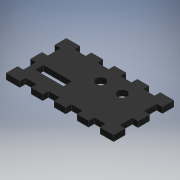
# Autodesk Inventor part: left
Saved by Autodesk Inventor 2019 (Build 230136000, 136)
## iProperties
Created: 2018-06-07
Part Number: left
Material: PBT Plastic Black
Document SubType Name: Modeling
Designer: stra92745
Density: 1.31 g/cm^3
Appearance: Smooth - White
Author: stra92745
Autodesk Inventor part; units mm, degrees
ref_plane "YZ Plane" through (0, 0, 0) normal (1, 0, 0) x (0, 1, 0)
ref_plane "XZ Plane" through (0, 0, 0) normal (0, 1, 0) x (-1, 0, 0)
ref_plane "XY Plane" through (0, 0, 0) normal (0, 0, 1) x (1, 0, 0)
sketch "Sketch1" plane through (0, 0, 0) normal (0, 1, 0) x (-1, 0, 0)
  line L0 (0, 0) -> (-75, 0)
  line L1 (-75, 0) -> (-75, -42)
  line L2 (-75, -42) -> (0, -42)
  line L3 (0, -42) -> (0, 0)
  line L4 (-8, -18) -> (-28, -18)
  line L5 (-28, -18) -> (-28, -12)
  line L6 (-28, -12) -> (-8, -12)
  line L7 (-8, -12) -> (-8, -18)
  circle A0 centre (-38, -28) radius 3.5
  circle A1 centre (-53, -28) radius 3.5
  dimension "d0" = 75
  dimension "d1" = 42
  dimension "d2" = 20
  dimension "d3" = 6
  dimension "d4" = 12
  dimension "d5" = 8
  dimension "d6" = 7
  dimension "d7" = 28
  dimension "d8" = 38
  dimension "d9" = 15
  constraints: 16 end point, 4 parallel, 2 centre point, 2 horizontal, 2 perpendicular, 1 equal radius, 1 horizontal alignment
  measures "d0" distance of L2.end L1.end
  measures "d1" distance of L1.end L0.end
  measures "d2" distance of L4.start L4.end
  measures "d3" distance of L4.end L5.end
  measures "d4" distance between parallel lines of L0 L6
  measures "d5" distance between parallel lines of L3 L7
  measures "d6" diameter of A0
  measures "d7" distance from line of L0 A0.centre
  measures "d8" distance from line of L3 A0.centre
  measures "d9" distance of A1.centre A0.centre
extrude "Extrusion1" add sketch "Sketch1" along normal blind 4
sketch "Sketch2" plane through (0, 4, 0) normal (0, 1, 0) x (1, 0, 0)
  line L0 (0, 42) -> (0, 0) construction
  line L1 (75, 42) -> (0, 42) construction
  line L2 (75, 0) -> (75, 42) construction
  line L3 (0, 0) -> (75, 0) construction
  line L4 (4, 38) -> (4, 4) construction
  line L5 (4, 4) -> (71, 4) construction
  line L6 (71, 4) -> (71, 38) construction
  line L7 (71, 38) -> (4, 38) construction
  line L8 (0, 42) -> (0, 0) construction
  line L9 (0, 21) -> (75, 21) construction
  line L10 (37.5, 42) -> (37.5, 0) construction
  line L11 (0, 34) -> (4, 34)
  line L12 (4, 34) -> (4, 25)
  line L13 (4, 25) -> (0, 25)
  line L14 (0, 25) -> (0, 34)
  line L15 (75, 42) -> (0, 42) projected
  line L16 (9.5, 38) -> (17.5, 38)
  line L17 (17.5, 38) -> (17.5, 42)
  line L18 (17.5, 42) -> (9.5, 42)
  line L19 (9.5, 42) -> (9.5, 38)
  line L20 (25.5, 38) -> (33.5, 38)
  line L21 (33.5, 38) -> (33.5, 42)
  line L22 (33.5, 42) -> (25.5, 42)
  line L23 (25.5, 42) -> (25.5, 38)
  line L24 (75, 34) -> (71, 34)
  line L25 (71, 34) -> (71, 25)
  line L26 (71, 25) -> (75, 25)
  line L27 (75, 25) -> (75, 34)
  line L28 (65.5, 38) -> (57.5, 38)
  line L29 (57.5, 38) -> (57.5, 42)
  line L30 (57.5, 42) -> (65.5, 42)
  line L31 (65.5, 42) -> (65.5, 38)
  line L32 (49.5, 38) -> (41.5, 38)
  line L33 (41.5, 38) -> (41.5, 42)
  line L34 (41.5, 42) -> (49.5, 42)
  line L35 (49.5, 42) -> (49.5, 38)
  line L36 (75, 0) -> (0, 0) construction
  line L37 (71, 4) -> (4, 4) construction
  line L38 (0, 8) -> (4, 8)
  line L39 (4, 8) -> (4, 17)
  line L40 (4, 17) -> (0, 17)
  line L41 (0, 17) -> (0, 8)
  line L42 (75, 0) -> (0, 0)
  line L43 (9.5, 4) -> (17.5, 4)
  line L44 (17.5, 4) -> (17.5, 0)
  line L45 (17.5, 0) -> (9.5, 0)
  line L46 (9.5, 0) -> (9.5, 4)
  line L47 (25.5, 4) -> (33.5, 4)
  line L48 (33.5, 4) -> (33.5, 0)
  line L49 (33.5, 0) -> (25.5, 0)
  line L50 (25.5, 0) -> (25.5, 4)
  line L51 (49.5, 4) -> (41.5, 4)
  line L52 (49.5, 0) -> (49.5, 4)
  line L53 (41.5, 0) -> (49.5, 0)
  line L54 (41.5, 4) -> (41.5, 0)
  line L55 (57.5, 4) -> (57.5, 0)
  line L56 (65.5, 4) -> (57.5, 4)
  line L57 (57.5, 0) -> (65.5, 0)
  line L58 (71, 8) -> (71, 17)
  line L59 (71, 17) -> (75, 17)
  line L60 (75, 17) -> (75, 8)
  line L61 (75, 8) -> (71, 8)
  line L62 (65.5, 0) -> (65.5, 4)
  dimension "d12" = 4
  dimension "d13" = 4
  dimension "d14" = 8
  dimension "d15" = 8
  dimension "d16" = 8
  dimension "d17" = 8
  dimension "d18" = 4
  constraints: 114 end point, 36 symmetric about line, 12 point on line, 4 midpoint, 4 parallel, 4 perpendicular, 2 horizontal, 1 collinear, 3 other
  measures "d12" distance between parallel lines of L1 L7
  measures "d13" distance between parallel lines of L9 L13
  measures "d14" distance between parallel lines of L11 L1
  measures "d15" distance of L20.start L20.end
  measures "d16" distance of L16.start L16.end
  measures "d17" distance between parallel lines of L23 L17
  measures "d18" distance between parallel lines of L10 L21
extrude "Extrusion2" cut sketch "Sketch2" against normal up to surface (4 mm away)
body "Solid1"
